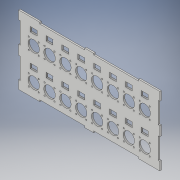
# Autodesk Inventor part: case_front
Saved by Autodesk Inventor 2019 (Build 230136000, 136)
## iProperties
Created: 2019-07-12
Part Number: case_front
Material: Generic
Document SubType Name: Modeling
Designer: Lino P
Density: 1 g/cm^3
Appearance: Default
Author: Lino P
Autodesk Inventor part; units mm, degrees
ref_plane "YZ Plane" through (0, 0, 0) normal (1, 0, 0) x (0, 1, 0)
ref_plane "XZ Plane" through (0, 0, 0) normal (0, 1, 0) x (-1, 0, 0)
ref_plane "XY Plane" through (0, 0, 0) normal (0, 0, 1) x (1, 0, 0)
sketch "Sketch1" plane through (0, 0, 0) normal (0, 0, 1) x (1, 0, 0)
  line L0 (0, 0) -> (27, 0)
  line L1 (27, 0) -> (27, 30.2)
  line L2 (27, 30.2) -> (0, 30.2)
  line L3 (0, 30.2) -> (0, 0)
  circle A0 centre (13.5, 15.1) radius 10.85
  circle A1 centre (4.1, 4.2) radius 1.3
  circle A2 centre (22.9, 26) radius 1.3
  line L4 (21.6, 26) -> (24.2, 26) construction
  line L5 (22.9, 26) -> (22.9, 27.3) construction
  line L6 (4.1, 4.2) -> (2.8, 4.2) construction
  line L7 (4.1, 4.2) -> (4.1, 2.9) construction
  line L8 (30, 0) -> (57, 0)
  line L9 (57, 0) -> (57, 30.2)
  line L10 (57, 30.2) -> (30, 30.2)
  line L11 (30, 30.2) -> (30, 0)
  circle A3 centre (43.5, 15.1) radius 10.85
  circle A4 centre (34.1, 4.2) radius 1.3
  circle A5 centre (52.9, 26) radius 1.3
  line L12 (51.6, 26) -> (54.2, 26) construction
  line L13 (52.9, 26) -> (52.9, 27.3) construction
  line L14 (34.1, 4.2) -> (32.8, 4.2) construction
  line L15 (34.1, 4.2) -> (34.1, 2.9) construction
  line L16 (60, 0) -> (87, 0)
  line L17 (87, 0) -> (87, 30.2)
  line L18 (87, 30.2) -> (60, 30.2)
  line L19 (60, 30.2) -> (60, 0)
  circle A6 centre (73.5, 15.1) radius 10.85
  circle A7 centre (64.1, 4.2) radius 1.3
  circle A8 centre (82.9, 26) radius 1.3
  line L20 (81.6, 26) -> (84.2, 26) construction
  line L21 (82.9, 26) -> (82.9, 27.3) construction
  line L22 (64.1, 4.2) -> (62.8, 4.2) construction
  line L23 (64.1, 4.2) -> (64.1, 2.9) construction
  line L24 (90, 0) -> (117, 0)
  line L25 (117, 0) -> (117, 30.2)
  line L26 (117, 30.2) -> (90, 30.2)
  line L27 (90, 30.2) -> (90, 0)
  circle A9 centre (103.5, 15.1) radius 10.85
  circle A10 centre (94.1, 4.2) radius 1.3
  circle A11 centre (112.9, 26) radius 1.3
  line L28 (111.6, 26) -> (114.2, 26) construction
  line L29 (112.9, 26) -> (112.9, 27.3) construction
  line L30 (94.1, 4.2) -> (92.8, 4.2) construction
  line L31 (94.1, 4.2) -> (94.1, 2.9) construction
  line L32 (120, 0) -> (147, 0)
  line L33 (147, 0) -> (147, 30.2)
  line L34 (147, 30.2) -> (120, 30.2)
  line L35 (120, 30.2) -> (120, 0)
  circle A12 centre (133.5, 15.1) radius 10.85
  circle A13 centre (124.1, 4.2) radius 1.3
  circle A14 centre (142.9, 26) radius 1.3
  line L36 (141.6, 26) -> (144.2, 26) construction
  line L37 (142.9, 26) -> (142.9, 27.3) construction
  line L38 (124.1, 4.2) -> (122.8, 4.2) construction
  line L39 (124.1, 4.2) -> (124.1, 2.9) construction
  line L40 (150, 0) -> (177, 0)
  line L41 (177, 0) -> (177, 30.2)
  line L42 (177, 30.2) -> (150, 30.2)
  line L43 (150, 30.2) -> (150, 0)
  circle A15 centre (163.5, 15.1) radius 10.85
  circle A16 centre (154.1, 4.2) radius 1.3
  circle A17 centre (172.9, 26) radius 1.3
  line L44 (171.6, 26) -> (174.2, 26) construction
  line L45 (172.9, 26) -> (172.9, 27.3) construction
  line L46 (154.1, 4.2) -> (152.8, 4.2) construction
  line L47 (154.1, 4.2) -> (154.1, 2.9) construction
  line L48 (180, 0) -> (207, 0)
  line L49 (207, 0) -> (207, 30.2)
  line L50 (207, 30.2) -> (180, 30.2)
  line L51 (180, 30.2) -> (180, 0)
  circle A18 centre (193.5, 15.1) radius 10.85
  circle A19 centre (184.1, 4.2) radius 1.3
  circle A20 centre (202.9, 26) radius 1.3
  line L52 (201.6, 26) -> (204.2, 26) construction
  line L53 (202.9, 26) -> (202.9, 27.3) construction
  line L54 (184.1, 4.2) -> (182.8, 4.2) construction
  line L55 (184.1, 4.2) -> (184.1, 2.9) construction
  line L56 (210, 0) -> (237, 0)
  line L57 (237, 0) -> (237, 30.2)
  line L58 (237, 30.2) -> (210, 30.2)
  line L59 (210, 30.2) -> (210, 0)
  circle A21 centre (223.5, 15.1) radius 10.85
  circle A22 centre (214.1, 4.2) radius 1.3
  circle A23 centre (232.9, 26) radius 1.3
  line L60 (231.6, 26) -> (234.2, 26) construction
  line L61 (232.9, 26) -> (232.9, 27.3) construction
  line L62 (214.1, 4.2) -> (212.8, 4.2) construction
  line L63 (214.1, 4.2) -> (214.1, 2.9) construction
  line L64 (0, -60) -> (27, -60)
  line L65 (27, -60) -> (27, -29.8)
  line L66 (27, -29.8) -> (0, -29.8)
  line L67 (0, -29.8) -> (0, -60)
  circle A24 centre (13.5, -44.9) radius 10.85
  circle A25 centre (4.1, -55.8) radius 1.3
  circle A26 centre (22.9, -34) radius 1.3
  line L68 (21.6, -34) -> (24.2, -34) construction
  line L69 (22.9, -34) -> (22.9, -32.7) construction
  line L70 (4.1, -55.8) -> (2.8, -55.8) construction
  line L71 (4.1, -55.8) -> (4.1, -57.1) construction
  line L72 (30, -60) -> (57, -60)
  line L73 (57, -60) -> (57, -29.8)
  line L74 (57, -29.8) -> (30, -29.8)
  line L75 (30, -29.8) -> (30, -60)
  circle A27 centre (43.5, -44.9) radius 10.85
  circle A28 centre (34.1, -55.8) radius 1.3
  circle A29 centre (52.9, -34) radius 1.3
  line L76 (51.6, -34) -> (54.2, -34) construction
  line L77 (52.9, -34) -> (52.9, -32.7) construction
  line L78 (34.1, -55.8) -> (32.8, -55.8) construction
  line L79 (34.1, -55.8) -> (34.1, -57.1) construction
  line L80 (60, -60) -> (87, -60)
  line L81 (87, -60) -> (87, -29.8)
  line L82 (87, -29.8) -> (60, -29.8)
  line L83 (60, -29.8) -> (60, -60)
  circle A30 centre (73.5, -44.9) radius 10.85
  circle A31 centre (64.1, -55.8) radius 1.3
  circle A32 centre (82.9, -34) radius 1.3
  line L84 (81.6, -34) -> (84.2, -34) construction
  line L85 (82.9, -34) -> (82.9, -32.7) construction
  line L86 (64.1, -55.8) -> (62.8, -55.8) construction
  line L87 (64.1, -55.8) -> (64.1, -57.1) construction
  line L88 (90, -60) -> (117, -60)
  line L89 (117, -60) -> (117, -29.8)
  line L90 (117, -29.8) -> (90, -29.8)
  line L91 (90, -29.8) -> (90, -60)
  circle A33 centre (103.5, -44.9) radius 10.85
  circle A34 centre (94.1, -55.8) radius 1.3
  circle A35 centre (112.9, -34) radius 1.3
  line L92 (111.6, -34) -> (114.2, -34) construction
  line L93 (112.9, -34) -> (112.9, -32.7) construction
  line L94 (94.1, -55.8) -> (92.8, -55.8) construction
  line L95 (94.1, -55.8) -> (94.1, -57.1) construction
  line L96 (120, -60) -> (147, -60)
  line L97 (147, -60) -> (147, -29.8)
  line L98 (147, -29.8) -> (120, -29.8)
  line L99 (120, -29.8) -> (120, -60)
  circle A36 centre (133.5, -44.9) radius 10.85
  circle A37 centre (124.1, -55.8) radius 1.3
  circle A38 centre (142.9, -34) radius 1.3
  line L100 (141.6, -34) -> (144.2, -34) construction
  line L101 (142.9, -34) -> (142.9, -32.7) construction
  line L102 (124.1, -55.8) -> (122.8, -55.8) construction
  line L103 (124.1, -55.8) -> (124.1, -57.1) construction
  line L104 (150, -60) -> (177, -60)
  line L105 (177, -60) -> (177, -29.8)
  line L106 (177, -29.8) -> (150, -29.8)
  line L107 (150, -29.8) -> (150, -60)
  circle A39 centre (163.5, -44.9) radius 10.85
  circle A40 centre (154.1, -55.8) radius 1.3
  circle A41 centre (172.9, -34) radius 1.3
  line L108 (171.6, -34) -> (174.2, -34) construction
  line L109 (172.9, -34) -> (172.9, -32.7) construction
  line L110 (154.1, -55.8) -> (152.8, -55.8) construction
  line L111 (154.1, -55.8) -> (154.1, -57.1) construction
  line L112 (180, -60) -> (207, -60)
  line L113 (207, -60) -> (207, -29.8)
  line L114 (207, -29.8) -> (180, -29.8)
  line L115 (180, -29.8) -> (180, -60)
  circle A42 centre (193.5, -44.9) radius 10.85
  circle A43 centre (184.1, -55.8) radius 1.3
  circle A44 centre (202.9, -34) radius 1.3
  line L116 (201.6, -34) -> (204.2, -34) construction
  line L117 (202.9, -34) -> (202.9, -32.7) construction
  line L118 (184.1, -55.8) -> (182.8, -55.8) construction
  line L119 (184.1, -55.8) -> (184.1, -57.1) construction
  line L120 (210, -60) -> (237, -60)
  line L121 (237, -60) -> (237, -29.8)
  line L122 (237, -29.8) -> (210, -29.8)
  line L123 (210, -29.8) -> (210, -60)
  circle A45 centre (223.5, -44.9) radius 10.85
  circle A46 centre (214.1, -55.8) radius 1.3
  circle A47 centre (232.9, -34) radius 1.3
  line L124 (231.6, -34) -> (234.2, -34) construction
  line L125 (232.9, -34) -> (232.9, -32.7) construction
  line L126 (214.1, -55.8) -> (212.8, -55.8) construction
  line L127 (214.1, -55.8) -> (214.1, -57.1) construction
  line L128 (-15, 60.2) -> (252, 60.2)
  line L129 (252, 60.2) -> (252, -70)
  line L130 (252, -70) -> (-15, -70)
  line L131 (-15, -70) -> (-15, 60.2)
  line L132 (7, 35.2) -> (20, 35.2)
  line L133 (20, 35.2) -> (20, 44.2)
  line L134 (20, 44.2) -> (7, 44.2)
  line L135 (7, 44.2) -> (7, 35.2)
  line L136 (7, 35.2) -> (20, 44.2) construction
  line L137 (20, 35.2) -> (7, 44.2) construction
  line L138 (50, 35.2) -> (50, 44.2)
  line L139 (37, 35.2) -> (50, 35.2)
  line L140 (50, 44.2) -> (37, 44.2)
  line L141 (50, 35.2) -> (37, 44.2) construction
  line L142 (37, 44.2) -> (37, 35.2)
  line L143 (37, 35.2) -> (50, 44.2) construction
  line L144 (80, 35.2) -> (80, 44.2)
  line L145 (67, 35.2) -> (80, 35.2)
  line L146 (80, 44.2) -> (67, 44.2)
  line L147 (80, 35.2) -> (67, 44.2) construction
  line L148 (67, 44.2) -> (67, 35.2)
  line L149 (67, 35.2) -> (80, 44.2) construction
  line L150 (110, 35.2) -> (110, 44.2)
  line L151 (97, 35.2) -> (110, 35.2)
  line L152 (110, 44.2) -> (97, 44.2)
  line L153 (110, 35.2) -> (97, 44.2) construction
  line L154 (97, 44.2) -> (97, 35.2)
  line L155 (97, 35.2) -> (110, 44.2) construction
  line L156 (140, 35.2) -> (140, 44.2)
  line L157 (127, 35.2) -> (140, 35.2)
  line L158 (140, 44.2) -> (127, 44.2)
  line L159 (140, 35.2) -> (127, 44.2) construction
  line L160 (127, 44.2) -> (127, 35.2)
  line L161 (127, 35.2) -> (140, 44.2) construction
  line L162 (170, 35.2) -> (170, 44.2)
  line L163 (157, 35.2) -> (170, 35.2)
  line L164 (170, 44.2) -> (157, 44.2)
  line L165 (170, 35.2) -> (157, 44.2) construction
  line L166 (157, 44.2) -> (157, 35.2)
  line L167 (157, 35.2) -> (170, 44.2) construction
  line L168 (200, 35.2) -> (200, 44.2)
  line L169 (187, 35.2) -> (200, 35.2)
  line L170 (200, 44.2) -> (187, 44.2)
  line L171 (200, 35.2) -> (187, 44.2) construction
  line L172 (187, 44.2) -> (187, 35.2)
  line L173 (187, 35.2) -> (200, 44.2) construction
  line L174 (230, 35.2) -> (230, 44.2)
  line L175 (217, 35.2) -> (230, 35.2)
  line L176 (230, 44.2) -> (217, 44.2)
  line L177 (230, 35.2) -> (217, 44.2) construction
  line L178 (217, 44.2) -> (217, 35.2)
  line L179 (217, 35.2) -> (230, 44.2) construction
  line L180 (20, -24.8) -> (20, -15.8)
  line L181 (7, -24.8) -> (20, -24.8)
  line L182 (20, -15.8) -> (7, -15.8)
  line L183 (20, -24.8) -> (7, -15.8) construction
  line L184 (7, -15.8) -> (7, -24.8)
  line L185 (7, -24.8) -> (20, -15.8) construction
  line L186 (50, -24.8) -> (50, -15.8)
  line L187 (37, -24.8) -> (50, -24.8)
  line L188 (50, -15.8) -> (37, -15.8)
  line L189 (50, -24.8) -> (37, -15.8) construction
  line L190 (37, -15.8) -> (37, -24.8)
  line L191 (37, -24.8) -> (50, -15.8) construction
  line L192 (80, -24.8) -> (80, -15.8)
  line L193 (67, -24.8) -> (80, -24.8)
  line L194 (80, -15.8) -> (67, -15.8)
  line L195 (80, -24.8) -> (67, -15.8) construction
  line L196 (67, -15.8) -> (67, -24.8)
  line L197 (67, -24.8) -> (80, -15.8) construction
  line L198 (110, -24.8) -> (110, -15.8)
  line L199 (97, -24.8) -> (110, -24.8)
  line L200 (110, -15.8) -> (97, -15.8)
  line L201 (110, -24.8) -> (97, -15.8) construction
  line L202 (97, -15.8) -> (97, -24.8)
  line L203 (97, -24.8) -> (110, -15.8) construction
  line L204 (140, -24.8) -> (140, -15.8)
  line L205 (127, -24.8) -> (140, -24.8)
  line L206 (140, -15.8) -> (127, -15.8)
  line L207 (140, -24.8) -> (127, -15.8) construction
  line L208 (127, -15.8) -> (127, -24.8)
  line L209 (127, -24.8) -> (140, -15.8) construction
  line L210 (170, -24.8) -> (170, -15.8)
  line L211 (157, -24.8) -> (170, -24.8)
  line L212 (170, -15.8) -> (157, -15.8)
  line L213 (170, -24.8) -> (157, -15.8) construction
  line L214 (157, -15.8) -> (157, -24.8)
  line L215 (157, -24.8) -> (170, -15.8) construction
  line L216 (200, -24.8) -> (200, -15.8)
  line L217 (187, -24.8) -> (200, -24.8)
  line L218 (200, -15.8) -> (187, -15.8)
  line L219 (200, -24.8) -> (187, -15.8) construction
  line L220 (187, -15.8) -> (187, -24.8)
  line L221 (187, -24.8) -> (200, -15.8) construction
  line L222 (230, -24.8) -> (230, -15.8)
  line L223 (217, -24.8) -> (230, -24.8)
  line L224 (230, -15.8) -> (217, -15.8)
  line L225 (230, -24.8) -> (217, -15.8) construction
  line L226 (217, -15.8) -> (217, -24.8)
  line L227 (217, -24.8) -> (230, -15.8) construction
  line L228 (-15, -4.9) -> (252, -4.9) construction
  line L229 (118.5, 60.2) -> (118.5, -70) construction
  line L230 (-15, 44.2) -> (-12, 44.2)
  line L231 (-12, 44.2) -> (-12, 4.2)
  line L232 (-12, 4.2) -> (-15, 4.2)
  line L233 (-15, 4.2) -> (-15, 44.2)
  line L234 (-15, -54) -> (-12, -54)
  line L235 (-12, -54) -> (-12, -14)
  line L236 (-12, -14) -> (-15, -14)
  line L237 (-15, -14) -> (-15, -54)
  line L238 (252, 44.2) -> (249, 44.2)
  line L239 (249, 44.2) -> (249, 4.2)
  line L240 (249, 4.2) -> (252, 4.2)
  line L241 (252, 4.2) -> (252, 44.2)
  line L242 (249, -54) -> (249, -14)
  line L243 (252, -54) -> (249, -54)
  line L244 (252, -14) -> (252, -54)
  line L245 (249, -14) -> (252, -14)
  line L246 (25, 60.2) -> (110, 60.2)
  line L247 (110, 60.2) -> (110, 57.2)
  line L248 (110, 57.2) -> (25, 57.2)
  line L249 (25, 57.2) -> (25, 60.2)
  line L250 (212, 60.2) -> (127, 60.2)
  line L251 (127, 60.2) -> (127, 57.2)
  line L252 (127, 57.2) -> (212, 57.2)
  line L253 (212, 57.2) -> (212, 60.2)
  line L254 (25, -70) -> (110, -70)
  line L255 (110, -70) -> (110, -67)
  line L256 (110, -67) -> (25, -67)
  line L257 (25, -67) -> (25, -70)
  line L258 (212, -67) -> (212, -70)
  line L259 (127, -70) -> (127, -67)
  line L260 (127, -67) -> (212, -67)
  line L261 (212, -70) -> (127, -70)
  line L262 (13.5, 30.2) -> (13.5, 0) construction
  line L263 (0, 15.1) -> (27, 15.1) construction
  circle A48 centre (4.1, 26) radius 1.3
  circle A49 centre (22.9, 4.2) radius 1.3
  circle A50 centre (34.1, 26) radius 1.3
  circle A51 centre (52.9, 4.2) radius 1.3
  circle A52 centre (64.1, 26) radius 1.3
  circle A53 centre (82.9, 4.2) radius 1.3
  circle A54 centre (94.1, 26) radius 1.3
  circle A55 centre (112.9, 4.2) radius 1.3
  circle A56 centre (124.1, 26) radius 1.3
  circle A57 centre (142.9, 4.2) radius 1.3
  circle A58 centre (154.1, 26) radius 1.3
  circle A59 centre (172.9, 4.2) radius 1.3
  circle A60 centre (184.1, 26) radius 1.3
  circle A61 centre (202.9, 4.2) radius 1.3
  circle A62 centre (214.1, 26) radius 1.3
  circle A63 centre (232.9, 4.2) radius 1.3
  circle A64 centre (4.1, -34) radius 1.3
  circle A65 centre (22.9, -55.8) radius 1.3
  circle A66 centre (34.1, -34) radius 1.3
  circle A67 centre (52.9, -55.8) radius 1.3
  circle A68 centre (64.1, -34) radius 1.3
  circle A69 centre (82.9, -55.8) radius 1.3
  circle A70 centre (94.1, -34) radius 1.3
  circle A71 centre (112.9, -55.8) radius 1.3
  circle A72 centre (124.1, -34) radius 1.3
  circle A73 centre (142.9, -55.8) radius 1.3
  circle A74 centre (154.1, -34) radius 1.3
  circle A75 centre (172.9, -55.8) radius 1.3
  circle A76 centre (184.1, -34) radius 1.3
  circle A77 centre (202.9, -55.8) radius 1.3
  circle A78 centre (214.1, -34) radius 1.3
  circle A79 centre (232.9, -55.8) radius 1.3
  point P0 (13.5, 39.7)
  point P1 (43.5, 39.7)
  point P2 (73.5, 39.7)
  point P3 (103.5, 39.7)
  point P4 (133.5, 39.7)
  point P5 (163.5, 39.7)
  point P6 (193.5, 39.7)
  point P7 (223.5, 39.7)
  point P8 (13.5, -20.3)
  point P9 (43.5, -20.3)
  point P10 (73.5, -20.3)
  point P11 (103.5, -20.3)
  point P12 (133.5, -20.3)
  point P13 (163.5, -20.3)
  point P14 (193.5, -20.3)
  point P15 (223.5, -20.3)
  dimension "d0" = 27
  dimension "d1" = 30.2
  dimension "d3" = 21.7
  dimension "d4" = 2.6
  dimension "d7" = 2.6
  dimension "d8" = 2.8
  dimension "d9" = 2.9
  dimension "d10" = 2.8
  dimension "d11" = 2.9
  dimension "d14" = 30
  dimension "d17" = 60
  dimension "d22" = 15
  dimension "d23" = 15
  dimension "d24" = 30
  dimension "d25" = 10
  dimension "d26" = 13
  dimension "d27" = 9
  dimension "d28" = 5
  dimension "d31" = 30
  dimension "d34" = 60
  dimension "d38" = 3
  dimension "d39" = 40
  dimension "d41" = 3
  dimension "d42" = 40
  dimension "d43" = 85
  dimension "d46" = 267
  dimension "d49" = 30
  dimension "d52" = 60
  constraints: 528 end point, 80 centre point, 80 point on circle, 39 midpoint, 26 symmetric about line, 10 parallel, 9 horizontal, 6 perpendicular, 4 vertical, 2 collinear, 2 point on line, 570 other
  measures "d0" distance of L2.end L1.end
  measures "d1" distance of L1.end L0.end
  measures "d3" diameter of A0
  measures "d4" diameter of A1
  measures "d7" diameter of A2
  measures "d8" distance from line of L1 L4.end
  measures "d9" distance from line of L2 L5.end
  measures "d10" distance from line of L3 L6.end
  measures "d11" distance from line of L0 L7.end
  measures "d14" distance of L1.end L9.end
  measures "d17" distance of L1.end L65.end
  measures "d22" distance between parallel lines of L131 L3
  measures "d23" distance between parallel lines of L57 L129
  measures "d24" distance between parallel lines of L18 L128
  measures "d25" distance between parallel lines of L72 L130
  measures "d26" distance of L134.end L133.end
  measures "d27" distance of L133.end L132.end
  measures "d28" distance between parallel lines of L2 L132
  measures "d31" distance of L132.end L138.start
  measures "d34" distance of L132.end L180.start
  measures "d38" distance of L231.end L232.end
  measures "d39" distance of L230.end L231.end
  measures "d41" distance of L246.end L247.end
  measures "d42" distance between parallel lines of L249 L131
  measures "d43" distance between parallel lines of L249 L247
  measures "d46" distance of L129.end L130.end
  measures "d49" distance of A48.centre A50.centre
  measures "d52" distance of A48.centre A64.centre
extrude "Extrusion2" add sketch "Sketch1" along normal blind 3 contours L3 L2 L1 L0 | L11 L10 L9 L8 | L19 L18 L17 L16 | L27 L26 L25 L24 | L35 L34 L33 L32 | L43 L42 L41 L40 | L51 L50 L49 L48 | L59 L58 L57 L56 | L67 L66 L65 L64 | L75 L74 L73 L72 | L83 L82 L81 L80 | L91 L90 L89 L88 | L99 L98 L97 L96 | L107 L106 L105 L104 | L115 L114 L113 L112 | L123 L122 L121 L120 | L128 L249 L248 L247 L251 L252 L253 L129 L238 L239 L240 L245 L242 L243 L130 L258 L260 L259 L255 L256 L257 L131 L234 L235 L236 L232 L231 L230
body "Solid2"
